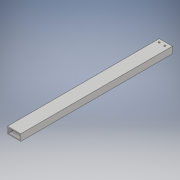
# Autodesk Inventor part: support beam 2
Saved by Autodesk Inventor 2017 (Build 210142000, 142)
## iProperties
Created: 2017-12-29
Part Number: support beam 2
Material: Generic
Document SubType Name: Modeling
Designer: Micah
Density: 1 g/cm^3
Appearance: Default
Author: Micah
Autodesk Inventor part; units mm, degrees
ref_plane "YZ Plane" through (0, 0, 0) normal (1, 0, 0) x (0, 1, 0)
ref_plane "XZ Plane" through (0, 0, 0) normal (0, 1, 0) x (-1, 0, 0)
ref_plane "XY Plane" through (0, 0, 0) normal (0, 0, 1) x (1, 0, 0)
sketch "Sketch1" plane through (0, 0, 0) normal (0, 0, 1) x (1, 0, 0)
  line L0 (0, 0) -> (50.8, 0)
  line L1 (50.8, 0) -> (50.8, -25.4)
  line L2 (50.8, -25.4) -> (0, -25.4)
  line L3 (0, -25.4) -> (0, 0)
  line L4 (3.175, -3.175) -> (47.625, -3.175)
  line L5 (47.625, -3.175) -> (47.625, -22.225)
  line L6 (47.625, -22.225) -> (3.175, -22.225)
  line L7 (3.175, -22.225) -> (3.175, -3.175)
  dimension "d0" = 50.8
  dimension "d1" = 25.4
  dimension "d2" = 44.45
  dimension "d3" = 19.05
  dimension "d4" = 3.175
  dimension "d5" = 3.175
  constraints: 16 end point, 4 parallel, 2 horizontal, 2 perpendicular
  measures "d0" distance of L1.end L2.end
  measures "d1" distance of L0.end L1.end
  measures "d2" distance of L5.end L6.end
  measures "d3" distance of L4.end L5.end
  measures "d4" distance between parallel lines of L4 L0
  measures "d5" distance between parallel lines of L7 L3
extrude "Extrusion1" add sketch "Sketch1" along normal blind 584.2
sketch "Sketch2" plane through (0, 0, 0) normal (0, 1, 0) x (1, 0, 0)
  circle A0 centre (12.7, -12.7) radius 3.175
  line L0 (3.175, 0) -> (47.625, 0) projected
  line L1 (23.7245, 0) -> (23.7245, -584.2)
  line L2 (47.625, -584.2) -> (3.175, -584.2) projected
  line L3 (23.7245, 0) -> (607.9245, 0) construction
  line L4 (0, 0) -> (0, -584.2) projected
  circle A1 centre (34.749, -12.7) radius 3.175
  line L5 (0, -311.15) -> (50.8388, -311.15)
  line L6 (47.625, 0) -> (47.625, -584.2) projected
  circle A2 centre (12.7, -609.6) radius 3.175
  circle A3 centre (34.749, -609.6) radius 3.175
  dimension "d8" = 6.35
  dimension "d9" = 90
  dimension "d10" = 12.7
  dimension "d11" = 12.7
  dimension "d12" = 311.15
  constraints: 6 end point, 4 centre point, 3 point on line, 3 symmetric about line, 2 perpendicular, 1 horizontal, 3 other
  measures "d8" diameter of A0
  measures "d9" angle of L1 L3
  measures "d10" distance from line of L0 A0.centre
  measures "d11" distance from line of L4 A0.centre
  measures "d12" distance between parallel lines of L0 L5
hole "Hole1" at (12.7, 0, 609.6) at (34.749, 0, 609.6) at (12.7, 0, 12.7) at (34.749, 0, 12.7) direction (0, -1, 0) diameter 6.35 depth 25.4 tip angle 118
body "Solid1"
